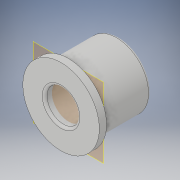
# Autodesk Inventor part: pvcconnector
Saved by Autodesk Inventor 2018 (Build 220112000, 112)
## iProperties
Created: 2019-05-01
Part Number: pvcconnector
Material: Generic
Document SubType Name: Modeling
Designer: F8PLTW
Density: 1 g/cm^3
Appearance: Default
Author: F8PLTW
Autodesk Inventor part; units mm, degrees
ref_plane "YZ Plane" through (0, 0, 0) normal (1, 0, 0) x (0, 1, 0)
ref_plane "XZ Plane" through (0, 0, 0) normal (0, 1, 0) x (-1, 0, 0)
ref_plane "XY Plane" through (0, 0, 0) normal (0, 0, 1) x (1, 0, 0)
sketch "Sketch1" plane through (0, 0, 0) normal (0, 0, 1) x (1, 0, 0)
  circle A0 centre (-5.0854, 2.5427) radius 10.795
  circle A1 centre (-5.0854, 2.5427) radius 21.082
  point P0 (0, 0)
  dimension "d0" = 21.59
  dimension "d1" = 42.164
  constraints: 2 centre point, 1 coincident
  measures "d0" diameter of A0
  measures "d1" diameter of A1
extrude "Extrusion1" add sketch "Sketch1" along normal blind 38.1
ref_plane "Work Plane1" through (-5.0854, 2.5427, 33.3375) normal (0, 0, 1) x (1, 0, 0)
sketch "Sketch2" plane through (-5.0854, 2.5427, 33.3375) normal (0, 0, 1) x (1, 0, 0)
  circle A0 centre (0, 0) radius 10.795
  circle A1 centre (0, 0) radius 25.1734
  point P0 (5.0854, -2.5427)
  constraints: 2 centre point, 1 coincident
extrude "Extrusion2" add sketch "Sketch2" along normal blind 4.7625
fillet "Fillet1" radius 1.5875 2 edges at (-15.8804, 2.5427, 38.1) (-26.1674, 2.5427, 0)
body "Solid1"
